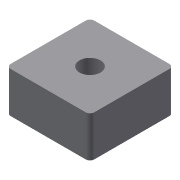
# Autodesk Inventor part: LG_G2_Lens
Saved by Autodesk Inventor 2019.4 (Build 234330000, 330)
## iProperties
Created: 2017-06-16
Part Number: LG_G2_Lens
Material: Generisch
Document SubType Name: Modeling
Designer: diederichbenedict
Density: 1 g/cm^3
Appearance: Vorgabe
Author: diederichbenedict
Autodesk Inventor part; units mm, degrees
ref_plane "YZ Plane" through (0, 0, 0) normal (1, 0, 0) x (0, 1, 0)
ref_plane "XZ Plane" through (0, 0, 0) normal (0, 1, 0) x (-1, 0, 0)
ref_plane "XY Plane" through (0, 0, 0) normal (0, 0, 1) x (1, 0, 0)
sketch "Skizze1" plane through (0, 0, 0) normal (0, 0, 1) x (1, 0, 0)
  line L0 (-4.865, 4.865) -> (4.865, 4.865)
  line L1 (4.865, 4.865) -> (4.865, -4.865)
  line L2 (4.865, -4.865) -> (-4.865, -4.865)
  line L3 (-4.865, -4.865) -> (-4.865, 4.865)
  line L4 (-4.865, 4.865) -> (4.865, -4.865) construction
  line L5 (4.865, 4.865) -> (-4.865, -4.865) construction
  circle A0 centre (0, 0) radius 1.2261
  dimension "d_1" = 9.73
  dimension "d1" = 9.73
  constraints: 12 end point, 2 midpoint, 2 parallel, 1 centre point, 1 coincident, 1 horizontal, 1 perpendicular
  measures "d_1" distance of L1.end L2.end
  measures "d1" distance of L0.end L1.end
extrude "Extrusion1" add sketch "Skizze1" along normal blind 4.74
fillet "Fillet1" radius 0.5 4 edges at (-4.865, -4.865, 2.37) (-4.865, 4.865, 2.37) (4.865, -4.865, 2.37) (4.865, 4.865, 2.37)
equation "\"d1\" = d_1"
